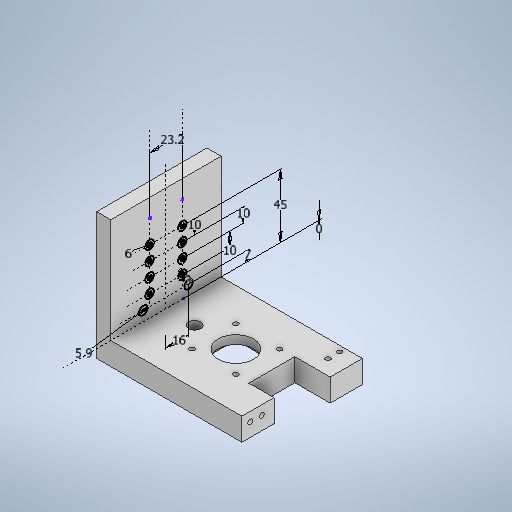
# Autodesk Inventor part: HolderV2
Saved by Autodesk Inventor 2025.1 (Build 291241000, 241)
## iProperties
Created: 2025-03-02
Part Number: HolderV2
Material: Generic
Document SubType Name: Modeling
Designer: 13156
Density: 1 g/cm^3
Appearance: Default
Author: 13156
Autodesk Inventor part; units mm, degrees
ref_plane "YZ Plane" through (0, 0, 0) normal (1, 0, 0) x (0, 1, 0)
ref_plane "XZ Plane" through (0, 0, 0) normal (0, 1, 0) x (-1, 0, 0)
ref_plane "XY Plane" through (0, 0, 0) normal (0, 0, 1) x (1, 0, 0)
sketch "Sketch1" plane through (0, 0, 0) normal (0, 1, 0) x (-1, 0, 0)
  line L0 (55, 39) -> (-55, 39)
  line L1 (-55, 39) -> (-55, -39)
  line L2 (-55, -39) -> (55, -39)
  line L3 (55, -39) -> (55, 39)
  line L4 (0, 0) -> (-9, 0) construction
  line L5 (0, 0) -> (0, -32.8738) construction
  circle A0 centre (-4.5, 0) radius 12.5
  line L6 (17, 21.5) -> (-26, 21.5)
  line L7 (-26, 21.5) -> (-26, -21.5)
  line L8 (-26, -21.5) -> (17, -21.5)
  line L9 (-55, 16.25) -> (-30, 16.25)
  line L10 (-30, 16.25) -> (-30, -16.25)
  line L11 (-30, -16.25) -> (-55, -16.25)
  line L12 (-55, -16.25) -> (-55, 16.25)
  circle A1 centre (-43, -26.7) radius 1.7
  circle A2 centre (-43, -35) radius 1.7
  line L13 (17, 21.5) -> (17, -21.5)
  circle A3 centre (24.64, 0) radius 4.2
  line L14 (-55, 39) -> (-47.75, 39)
  line L15 (-47.75, 39) -> (-47.75, 16.25)
  line L16 (-47.75, 16.25) -> (-55, 16.25)
  line L17 (-55, 16.25) -> (-55, 39)
  line L18 (-4.5, 0) -> (60.8131, 0) construction
  circle A4 centre (11, 15.5) radius 1.7
  circle A5 centre (11, -15.5) radius 1.7
  circle A6 centre (-20, -15.5) radius 1.7
  circle A7 centre (-20, 15.5) radius 1.7
  line L19 (-20, 15.5) -> (28.84, 15.5) construction
  line L20 (-20, 15.5) -> (-20, -27.9824) construction
  line L21 (-20, -15.5) -> (11, -15.5) construction
  line L22 (11, -15.5) -> (11, 26.1291) construction
  line L23 (-43, -26.7) -> (-43, -54.4551) construction
  line L24 (55, 39) -> (45, 39)
  line L25 (45, 39) -> (45, -39)
  line L26 (45, -39) -> (55, -39)
  line L27 (55, -39) -> (55, 39)
  point P0 (-55, 27.625)
  point P1 (-47.75, 27.625)
  point P2 (-42.5, -16.25)
  point P3 (-42.5, 16.25)
  point P4 (55, 0)
  dimension "d0" = 78
  dimension "d1" = 110
  dimension "d2" = 7.25
  dimension "d3" = 25
  dimension "d4" = 32.5
  dimension "d5" = 25
  dimension "d6" = 43
  dimension "d7" = 21.5
  dimension "d8" = 8.4
  dimension "d9" = 30.36
  dimension "d10" = 4
  dimension "d11" = 3.4
  dimension "d12" = 6
  dimension "d13" = 6
  dimension "d14" = 6
  dimension "d15" = 6
  dimension "d16" = 3.4
  dimension "d17" = 4
  dimension "d18" = 8.3
  dimension "d19" = 13
  dimension "d20" = 13
  dimension "d21" = 10
  constraints: 56 end point, 9 horizontal, 9 parallel, 8 centre point, 8 perpendicular, 7 point on line, 6 midpoint, 4 equal radius, 3 vertical, 1 coincident, 4 other
  measures "d0" distance of L2.end L0.start
  measures "d1" distance of L1.end L2.end
  measures "d2" distance of point (-55, 27.625) point (-47.75, 27.625)
  measures "d3" distance between parallel lines of L1 L10
  measures "d4" distance of point (-42.5, -16.25) point (-42.5, 16.25)
  measures "d5" diameter of A0
  measures "d6" distance of L6.start L8.end
  measures "d7" distance from line of L13 L18.start
  measures "d8" diameter of A3
  measures "d9" distance of point (55, 0) A3.centre
  measures "d10" distance between parallel lines of L10 L7
  measures "d11" diameter of A4
  measures "d12" distance from line of L6 L19.start
  measures "d13" distance from line of L7 L19.start
  measures "d14" distance from line of L13 L21.end
  measures "d15" distance between parallel lines of L8 L21
  measures "d16" diameter of A1
  measures "d17" distance from line of L2 A2.centre
  measures "d18" distance of L23.start A2.centre
  measures "d19" distance from line of L10 L23.start
  measures "d20" distance from line of L10 A2.centre
  measures "d21" distance between parallel lines of L27 L25
extrude "Extrusion1" add sketch "Sketch1" along normal blind 16 contours L3 L2 L25 L0 | L25 L2 L1 L11 L10 L9 L15 L0 | L13 L8 L7 L6
extrude "Extrusion2" add sketch "Sketch1" along normal blind 90 contours L3 L2 L25 L0
ref_plane "Work Plane1" through (0, 10, 0) normal (0, -1, 0) x (1, 0, 0)
extrude "Extrusion3" cut sketch "Sketch1" along normal up to surface (10 mm away) contours A0 | L13 L8 L7 L6 | A4 | A5 | A6 | A7
sketch "Sketch2" plane through (47.75, 0, 39) normal (1, 0, 0) x (0, 0, -1)
  circle A0 centre (5.925, 9.5) radius 1.7
  circle A1 centre (14.225, 9.5) radius 1.7
  line L0 (0, 16) -> (22.75, 16) projected
  line L1 (5.925, 9.5) -> (23.5795, 9.5) construction
  line L2 (0, 0) -> (0, 16) construction
  point P0 (39, 0)
  point P1 (0, 8)
  dimension "d29" = 3.4
  dimension "d30" = 6.5
  dimension "d31" = 8.3
  dimension "d32" = 5.925
  constraints: 2 centre point, 2 end point, 1 equal radius, 1 horizontal, 1 midpoint, 1 point on line
  measures "d29" diameter of A0
  measures "d30" distance from line of L0 L1.start
  measures "d31" distance of L1.start A1.centre
  measures "d32" horizontal distance of point (0, 8) L1.start
extrude "Extrusion4" cut sketch "Sketch2" against normal blind 8
sketch "Sketch3" plane through (-45, 16, -39) normal (1, 0, 0) x (0, 0, -1)
  circle A0 centre (-55, 7) radius 2.95
  circle A1 centre (-23, 7) radius 2.95
  circle A2 centre (-50.6, 45) radius 1.5
  circle A3 centre (-27.4, 45) radius 1.5
  circle A4 centre (-50.6, 35) radius 1.5
  circle A5 centre (-27.4, 35) radius 1.5
  circle A6 centre (-50.6, 25) radius 1.5
  circle A7 centre (-27.4, 25) radius 1.5
  circle A8 centre (-50.6, 15) radius 1.5
  circle A9 centre (-27.4, 15) radius 1.5
  line L0 (-111.9062, 0) -> (57.702, 0) construction
  line L1 (-39, -16) -> (-39, 89.2997) construction
  line L2 (-50.6, 115.8205) -> (-50.6, 7.4017) construction
  line L3 (-27.4, 116.2222) -> (-27.4, 7) construction
  line L4 (-22.75, 0) -> (0, 0) construction
  line L5 (-23, 7) -> (-72.4009, 7) construction
  line L6 (-27.4, 45) -> (-61.2573, 45) construction
  line L7 (-27.4, 35) -> (-63.1607, 35) construction
  line L8 (-27.4, 25) -> (-66.8484, 25) construction
  line L9 (-27.4, 15) -> (-66.8484, 15) construction
  circle A10 centre (-27.4, 45) radius 3
  circle A11 centre (-27.4, 35) radius 3
  circle A12 centre (-27.4, 25) radius 3
  circle A13 centre (-27.4, 15) radius 3
  circle A14 centre (-50.6, 15) radius 3
  circle A15 centre (-50.6, 25) radius 3
  circle A16 centre (-50.6, 35) radius 3
  circle A17 centre (-50.6, 45) radius 3
  point P0 (-27.4, 61.6111)
  point P1 (-50.6, 61.6111)
  point P2 (-27.1021, 0)
  dimension "d35" = 5.9
  dimension "d36" = 0
  dimension "d37" = 7
  dimension "d38" = 16
  dimension "d39" = 23.2
  dimension "d40" = 3
  dimension "d41" = 10
  dimension "d42" = 45
  dimension "d43" = 10
  dimension "d44" = 10
  dimension "d45" = 6
  constraints: 18 centre point, 18 end point, 15 equal radius, 14 point on line, 8 coincident, 6 horizontal, 3 midpoint, 3 vertical, 1 perpendicular, 1 symmetric about line, 1 other
  measures "d35" diameter of A0
  measures "d36" distance between parallel lines of L4 L0
  measures "d37" distance from line of L5.start L4
  measures "d38" distance from line of L1 L5.start
  measures "d39" distance of point (-27.4, 61.611) point (-50.6, 61.611)
  measures "d40" diameter of A9
  measures "d41" distance of L7.start L6.start
  measures "d42" vertical distance of point (-27.102, 0) L6.start
  measures "d43" distance of L8.start L7.start
  measures "d44" distance of L8.start L9.start
  measures "d45" diameter of A17
equation "\"d14\" = d13"
equation "\"d15\" = d13"
equation "\"d20\" = d19"
body "Solid1"
